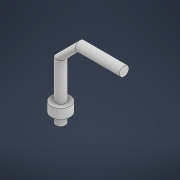
# Autodesk Inventor part: gud gear stand proto 1 2
Saved by Autodesk Inventor 2021 (Build 250183000, 183)
## iProperties
Created: 2021-02-08
Part Number: gud gear stand proto 1 2
Material: Generic
Document SubType Name: Modeling
Designer: benji
Density: 1 g/cm^3
Appearance: Default
Author: benji
Autodesk Inventor part; units mm, degrees
ref_plane "XZ Plane" through (0, 0, 0) normal (0, 1, 0) x (-1, 0, 0)
ref_plane "XY Plane" through (0, 0, 0) normal (0, 0, 1) x (1, 0, 0)
sketch "Sketch1" plane through (0, 0, 0) normal (0, 1, 0) x (-1, 0, 0)
  circle A0 centre (0, 0) radius 5
  dimension "d0" = 10
  constraints: 1 centre point, 1 coincident
  measures "d0" diameter of A0
extrude "Extrusion1" add sketch "Sketch1" along normal blind 5
sketch "Sketch2" plane through (0, 0, 0) normal (0, -1, 0) x (1, 0, 0)
  circle A0 centre (0, 0) radius 2.5
  dimension "d3" = 5
  constraints: 1 centre point, 1 coincident
  measures "d3" diameter of A0
extrude "Extrusion2" add sketch "Sketch2" along normal blind 5
sketch "Sketch3" plane through (0, 5, 0) normal (0, 1, 0) x (1, 0, 0)
  circle A0 centre (0, 0) radius 2.5
  dimension "d6" = 5
  constraints: 1 centre point, 1 coincident
  measures "d6" diameter of A0
extrude "Extrusion3" add sketch "Sketch3" along normal blind 20
ref_plane "Work Plane1" through (15, 0, 0) normal (1, 0, 0) x (0, 1, 0)
sketch "Sketch6" plane through (15, 0, 0) normal (1, 0, 0) x (0, 1, 0)
  line L0 (25, -2.5) -> (25, 2.5) projected
  line L1 (25, 0) -> (40.064, 0)
  line L2 (40.064, 0) -> (40.064, 4.909)
  circle A0 centre (40.064, 4.909) radius 2.5
  point P0 (0, 0)
  dimension "d28" = 15.064
  dimension "d29" = 4.909
  dimension "d30" = 5
  constraints: 4 end point, 1 centre point, 1 coincident, 1 horizontal, 1 midpoint, 1 perpendicular
  measures "d28" distance of L1.start L1.end
  measures "d29" distance of L1.end L2.end
  measures "d30" diameter of A0
extrude "Extrusion6" add sketch "Sketch6" along normal blind 25
loft "Loft3" add section 1 edges at (-2.5, 25, 0) section 2 edges at (15, 37.564, 4.909)
sketch "Sketch7" plane through (40, 40.064, 4.909) normal (1, 0, 0) x (0, 0, -1)
  circle A0 centre (0, 0) radius 2.5
  point P0 (4.909, -40.064)
  dimension "d37" = 5
  constraints: 1 centre point
  measures "d37" diameter of A0
extrude "Extrusion7" cut sketch "Sketch7" against normal blind 1.733
body "Solid1"
